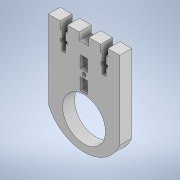
# Autodesk Inventor part: Крепление_мотора2_платформа
Saved by Autodesk Inventor 2020 (Build 240168000, 168)
## iProperties
Created: 2022-02-01
Part Number: Крепление_мотора2_платформа
Material: Типовые
Document SubType Name: Modeling
Designer: Администратор
Density: 1 g/cm^3
Appearance: По умолчанию
Autodesk Inventor part; units mm, degrees
ref_plane "YZ Plane" through (0, 0, 0) normal (1, 0, 0) x (0, 1, 0)
ref_plane "XZ Plane" through (0, 0, 0) normal (0, 1, 0) x (-1, 0, 0)
ref_plane "XY Plane" through (0, 0, 0) normal (0, 0, 1) x (1, 0, 0)
sketch "0" plane through (0, 0, 0) normal (0, 0, 1) x (1, 0, 0)
  line L0 (4, 55.5) -> (4, 61.5)
  line L1 (4, 61.5) -> (14, 61.5)
  line L2 (14, 61.5) -> (14, 55.5)
  line L3 (20, 55.5) -> (18.5, 55.5)
  line L4 (18.5, 55.5) -> (18.5, 49.25)
  line L5 (18.5, 40.5) -> (15.5, 40.5)
  line L6 (15.5, 40.5) -> (15.5, 46.75)
  line L7 (14.25, 49.25) -> (15.5, 49.25)
  line L8 (19.75, 49.25) -> (19.75, 46.75)
  line L9 (19.75, 46.75) -> (18.5, 46.75)
  line L10 (14.25, 46.75) -> (14.25, 49.25)
  line L11 (15.5, 49.25) -> (15.5, 55.5)
  line L12 (15.5, 46.75) -> (14.25, 46.75)
  line L13 (18.5, 49.25) -> (19.75, 49.25)
  line L14 (15.5, 55.5) -> (14, 55.5)
  line L15 (20, 61.5) -> (30, 61.5)
  line L16 (20, 55.5) -> (20, 61.5)
  line L17 (18.5, 46.75) -> (18.5, 40.5)
  line L18 (-30, 61.5) -> (-20, 61.5)
  line L19 (-20, 61.5) -> (-20, 55.5)
  line L20 (-14, 55.5) -> (-15.5, 55.5)
  line L21 (-15.5, 55.5) -> (-15.5, 49.25)
  line L22 (-15.5, 40.5) -> (-18.5, 40.5)
  line L23 (-18.5, 40.5) -> (-18.5, 46.75)
  line L24 (-19.75, 49.25) -> (-18.5, 49.25)
  line L25 (-14.25, 49.25) -> (-14.25, 46.75)
  line L26 (-14.25, 46.75) -> (-15.5, 46.75)
  line L27 (-19.75, 46.75) -> (-19.75, 49.25)
  line L28 (-18.5, 49.25) -> (-18.5, 55.5)
  line L29 (-18.5, 46.75) -> (-19.75, 46.75)
  line L30 (-15.5, 49.25) -> (-14.25, 49.25)
  line L31 (-18.5, 55.5) -> (-20, 55.5)
  line L32 (-14, 61.5) -> (-4, 61.5)
  line L33 (-14, 55.5) -> (-14, 61.5)
  line L34 (-4, 61.5) -> (-4, 55.5)
  line L35 (-15.5, 46.75) -> (-15.5, 40.5)
  line L36 (-3, 55.5) -> (-4, 55.5)
  line L37 (3, 55.5) -> (4, 55.5)
  line L38 (30, 61.5) -> (30, 55.5)
  circle A0 centre (0, 0) radius 18
  line L39 (30, 55.5) -> (30, -4)
  line L40 (-30, -4) -> (-30, 61.5)
  arc A1 (-30, -4) -> (30, -4) centre (0, 8.5) ccw
  line L41 (-3, 19.5) -> (-3, 29.5)
  line L42 (-3, 29.5) -> (3, 29.5)
  line L43 (3, 29.5) -> (3, 19.5)
  line L44 (3, 19.5) -> (-3, 19.5)
  line L45 (-3, 35.5) -> (-3, 45.5)
  line L46 (3, 45.5) -> (3, 35.5)
  line L47 (3, 35.5) -> (-3, 35.5)
  circle A2 centre (0, 32.5) radius 1.6
  line L48 (-3, 45.5) -> (3, 45.5)
  line L49 (-3, 55.5) -> (3, 55.5)
  point P0 (-30, -4)
  point P1 (30, -4)
  constraints: 100 end point, 3 centre point, 2 point on circle
sketch "Эскиз3" plane through (0, 0, 0) normal (0, 0, 1) x (1, 0, 0)
  circle A0 centre (0, 0) radius 18 projected
  circle A1 centre (0, 32.5) radius 1.6 projected
  line L0 (30, 55.5) -> (30, -4) projected
  line L1 (-30, -4) -> (-30, 61.5) projected
  line L2 (-30, 61.5) -> (-20, 61.5) projected
  line L3 (30, 61.5) -> (30, 55.5) projected
  line L4 (20, 61.5) -> (30, 61.5) projected
  line L5 (20, 55.5) -> (20, 61.5) projected
  line L6 (20, 55.5) -> (18.5, 55.5) projected
  line L7 (18.5, 55.5) -> (18.5, 49.25) projected
  line L8 (18.5, 49.25) -> (19.75, 49.25) projected
  line L9 (19.75, 49.25) -> (19.75, 46.75) projected
  line L10 (19.75, 46.75) -> (18.5, 46.75) projected
  line L11 (18.5, 46.75) -> (18.5, 40.5) projected
  line L12 (18.5, 40.5) -> (15.5, 40.5) projected
  line L13 (15.5, 40.5) -> (15.5, 46.75) projected
  line L14 (15.5, 46.75) -> (14.25, 46.75) projected
  line L15 (14.25, 46.75) -> (14.25, 49.25) projected
  line L16 (14.25, 49.25) -> (15.5, 49.25) projected
  line L17 (15.5, 49.25) -> (15.5, 55.5) projected
  line L18 (15.5, 55.5) -> (14, 55.5) projected
  line L19 (4, 61.5) -> (14, 61.5) projected
  line L20 (4, 55.5) -> (4, 61.5) projected
  line L21 (-3, 55.5) -> (3, 55.5) projected
  line L22 (3, 55.5) -> (4, 55.5) projected
  line L23 (14, 61.5) -> (14, 55.5) projected
  line L24 (-14, 61.5) -> (-4, 61.5) projected
  line L25 (-4, 61.5) -> (-4, 55.5) projected
  line L26 (-14, 55.5) -> (-15.5, 55.5) projected
  line L27 (-15.5, 55.5) -> (-15.5, 49.25) projected
  line L28 (-18.5, 49.25) -> (-18.5, 55.5) projected
  line L29 (-18.5, 55.5) -> (-20, 55.5) projected
  line L30 (-20, 61.5) -> (-20, 55.5) projected
  line L31 (-19.75, 49.25) -> (-18.5, 49.25) projected
  line L32 (-19.75, 46.75) -> (-19.75, 49.25) projected
  line L33 (-18.5, 46.75) -> (-19.75, 46.75) projected
  line L34 (-18.5, 40.5) -> (-18.5, 46.75) projected
  line L35 (-15.5, 40.5) -> (-18.5, 40.5) projected
  line L36 (-15.5, 46.75) -> (-15.5, 40.5) projected
  line L37 (-14.25, 46.75) -> (-15.5, 46.75) projected
  line L38 (-14.25, 49.25) -> (-14.25, 46.75) projected
  line L39 (-15.5, 49.25) -> (-14.25, 49.25) projected
  arc A2 (-30, -4) -> (30, -4) centre (0, 8.5) ccw projected
  line L40 (3, 29.5) -> (3, 19.5) projected
  line L41 (-3, 29.5) -> (3, 29.5) projected
  circle A3 centre (0, 0) radius 18
  circle A4 centre (0, 32.5) radius 1.6
  line L42 (-3, 45.5) -> (3, 45.5)
  line L43 (3, 45.5) -> (3, 35.5)
  line L44 (3, 35.5) -> (-3, 35.5)
  line L45 (-3, 35.5) -> (-3, 45.5)
  line L46 (-3, 29.5) -> (3, 29.5)
  line L47 (3, 29.5) -> (3, 19.5)
  line L48 (3, 19.5) -> (-3, 19.5)
  line L49 (-3, 19.5) -> (-3, 29.5)
  line L50 (18.5, 40.5) -> (15.5, 40.5)
  line L51 (15.5, 40.5) -> (15.5, 46.75)
  line L52 (18.5, 46.75) -> (18.5, 40.5)
  line L53 (19.75, 49.25) -> (19.75, 46.75)
  line L54 (14.25, 46.75) -> (14.25, 49.25)
  line L55 (18.5, 55.5) -> (18.5, 49.25)
  line L56 (15.5, 49.25) -> (15.5, 55.5)
  line L57 (20, 61.5) -> (20, 55.5)
  line L58 (14, 55.5) -> (14, 61.5)
  line L59 (4, 55.5) -> (-4, 55.5)
  line L60 (-4, 55.5) -> (-4, 61.5)
  line L61 (4, 61.5) -> (4, 55.5)
  line L62 (-20, 55.5) -> (-20, 61.5)
  line L63 (-14, 61.5) -> (-14, 55.5)
  line L64 (-15.5, 55.5) -> (-15.5, 49.25)
  line L65 (-18.5, 49.25) -> (-18.5, 55.5)
  line L66 (-14.25, 49.25) -> (-14.25, 46.75)
  line L67 (-19.75, 46.75) -> (-19.75, 49.25)
  line L68 (-15.5, 46.75) -> (-15.5, 40.5)
  line L69 (-15.5, 40.5) -> (-18.5, 40.5)
  line L70 (-18.5, 40.5) -> (-18.5, 46.75)
  line L71 (-14, 55.5) -> (-15.5, 55.5)
  line L72 (-18.5, 55.5) -> (-20, 55.5)
  line L73 (-19.75, 49.25) -> (-18.5, 49.25)
  line L74 (-15.5, 49.25) -> (-14.25, 49.25)
  line L75 (-14.25, 46.75) -> (-15.5, 46.75)
  line L76 (-18.5, 46.75) -> (-19.75, 46.75)
  line L77 (20, 55.5) -> (18.5, 55.5)
  line L78 (15.5, 55.5) -> (14, 55.5)
  line L79 (14.25, 49.25) -> (15.5, 49.25)
  line L80 (18.5, 49.25) -> (19.75, 49.25)
  line L81 (19.75, 46.75) -> (18.5, 46.75)
  line L82 (15.5, 46.75) -> (14.25, 46.75)
  line L83 (-30, 61.5) -> (-20, 61.5)
  line L84 (-14, 61.5) -> (-4, 61.5)
  line L85 (20, 61.5) -> (30, 61.5)
  line L86 (14, 61.5) -> (4, 61.5)
  line L87 (30, 61.5) -> (30, -4)
  line L88 (-30, -4) -> (-30, 61.5)
  arc A5 (-30, -4) -> (30, -4) centre (0, 8.5) ccw
  point P0 (0, 0)
  constraints: 94 end point, 24 equal length, 11 perpendicular, 10 horizontal, 3 centre point, 3 concentric, 2 coincident, 2 point on circle
extrude "Выдавливание2" add sketch "Эскиз3" along normal blind 10
